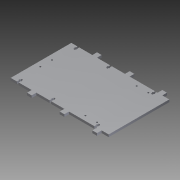
# Autodesk Inventor part: pieza central base superior
Saved by Autodesk Inventor 2012 SP1 (Build 160190100, 190)
## iProperties
Created: 2014-12-27
Part Number: pieza central base superior
Material: Default
Document SubType Name: Modeling
Designer: PRINCIPAL
Density: 1 g/cm^3
Author: PRINCIPAL
Autodesk Inventor part; units mm, degrees
ref_plane "YZ Plane" through (0, 0, 0) normal (1, 0, 0) x (0, 1, 0)
ref_plane "XZ Plane" through (0, 0, 0) normal (0, 1, 0) x (-1, 0, 0)
ref_plane "XY Plane" through (0, 0, 0) normal (0, 0, 1) x (1, 0, 0)
sketch "Boceto1" plane through (0, 0, 0) normal (0, 0, 1) x (1, 0, 0)
  line L0 (0, 0) -> (195, 0)
  line L1 (195, 0) -> (195, -130)
  line L2 (195, -130) -> (0, -130)
  line L3 (-15, 0) -> (-15, -130)
  line L4 (0, -130) -> (-15, -130)
  line L5 (0, 0) -> (-15, 0)
  dimension "d1" = 130
  constraints: 12 end point, 2 parallel, 2 perpendicular, 1 horizontal
  measures "d1" distance between parallel lines of L2 L0
extrude "Extrusión1" add sketch "Boceto1" along normal blind 5
sketch "Boceto2" plane through (0, 0, 5) normal (0, 0, 1) x (1, 0, 0)
  line L0 (-15, 0) -> (195, 0) projected
  line L1 (195, -130) -> (-15, -130) projected
  line L2 (30, 0) -> (40, 0)
  line L3 (100, 0) -> (110, 0)
  line L4 (170, 0) -> (180, 0)
  line L5 (170, -130) -> (180, -130)
  line L6 (100, -130) -> (110, -130)
  line L7 (30, -130) -> (40, -130)
  line L8 (40, 5) -> (40, 0)
  line L9 (40, -130) -> (40, -135)
  line L10 (30, -135) -> (30, -130)
  line L11 (30, 0) -> (30, 5)
  line L12 (110, 5) -> (110, 0)
  line L13 (110, -130) -> (110, -135)
  line L14 (100, -135) -> (100, -130)
  line L15 (100, 0) -> (100, 5)
  line L16 (180, 5) -> (180, 0)
  line L17 (180, -130) -> (180, -135)
  line L18 (170, -135) -> (170, -130)
  line L19 (170, 0) -> (170, 5)
  line L20 (30, 5) -> (30, 10)
  line L21 (40, 10) -> (40, 5)
  line L22 (100, 5) -> (100, 10)
  line L23 (110, 10) -> (110, 5)
  line L24 (170, 5) -> (170, 10)
  line L25 (180, 10) -> (180, 5)
  line L26 (40, -135) -> (40, -140)
  line L27 (30, -140) -> (30, -135)
  line L28 (110, -135) -> (110, -140)
  line L29 (100, -140) -> (100, -135)
  line L30 (180, -135) -> (180, -140)
  line L31 (170, -140) -> (170, -135)
  line L32 (170, 10) -> (180, 10)
  line L33 (30, 10) -> (40, 10)
  line L34 (100, 10) -> (110, 10)
  line L35 (180, -140) -> (170, -140)
  line L36 (110, -140) -> (100, -140)
  line L37 (40, -140) -> (30, -140)
  constraints: 72 end point, 27 perpendicular, 24 equal length, 12 point on line
extrude "Extrusión2" add sketch "Boceto2" against normal blind 5
sketch "Boceto3" plane through (0, 0, 5) normal (0, 0, 1) x (1, 0, 0)
  line L0 (195, 0) -> (195, -130) projected
  line L1 (180, 0) -> (195, 0) projected
  line L2 (-15, -130) -> (-15, 0) projected
  circle A0 centre (135, -120) radius 1.75
  circle A1 centre (160, -120) radius 1.75
  circle A2 centre (135, -10) radius 1.75
  circle A3 centre (160, -10) radius 1.75
  circle A4 centre (-4, -52.5) radius 1.75
  circle A5 centre (-4, -77.5) radius 1.75
  point P0 (30, 0)
  point P1 (30, -130)
  point P2 (0, 0)
  dimension "d20" = 3.5
  dimension "d21" = 3.5
  dimension "d22" = 3.5
  dimension "d23" = 3.5
  dimension "d24" = 3.5
  dimension "d25" = 3.5
  dimension "d26" = 25
  dimension "d27" = 25
  dimension "d28" = 25
  dimension "d29" = 10
  dimension "d30" = 10
  dimension "d31" = 150
  dimension "d32" = 150
  dimension "d33" = 52.5
  dimension "d34" = 199
  constraints: 6 centre point
  measures "d20" diameter of A0
  measures "d21" diameter of A1
  measures "d22" diameter of A2
  measures "d23" diameter of A3
  measures "d24" diameter of A4
  measures "d25" diameter of A5
  measures "d26" distance of A3.centre A2.centre
  measures "d27" distance of A1.centre A0.centre
  measures "d28" distance of A4.centre A5.centre
  measures "d29" vertical distance of A2.centre point (30, 0)
  measures "d30" vertical distance of point (30, -130) A0.centre
  measures "d31" distance from line of A0.centre L2
  measures "d32" distance from line of L2 A2.centre
  measures "d33" distance from line of A4.centre L1
  measures "d34" distance from line of L0 A4.centre
extrude "Extrusión3" cut sketch "Boceto3" against normal blind 10
sketch "Boceto4" plane through (0, 0, 5) normal (0, 0, 1) x (1, 0, 0)
  line L0 (-1.6674, -130.3426) -> (-1.6674, -125.4313)
  line L1 (1.8326, -130.3426) -> (-1.6674, -130.3426)
  line L2 (1.8326, -125.4313) -> (1.8326, -130.3426)
  line L3 (-1.6674, -125.4313) -> (-2.6674, -125.4313)
  line L4 (-2.6674, -123.0313) -> (-1.6674, -123.0313)
  line L5 (-1.6674, -123.0313) -> (-1.6674, -120.2573)
  line L6 (1.8326, -120.2573) -> (1.8326, -123.0313)
  line L7 (2.8326, -125.4313) -> (1.8326, -125.4313)
  line L8 (2.8326, -123.0313) -> (2.8326, -125.4313)
  line L9 (1.8326, -123.0313) -> (2.8326, -123.0313)
  line L10 (1.8326, -120.2573) -> (-1.6674, -120.2573)
  line L11 (-2.6674, -125.4313) -> (-2.6674, -123.0313)
  line L12 (167.9972, -120.715) -> (164.4972, -120.715)
  line L13 (167.9972, -120.715) -> (167.9972, -123.4891)
  line L14 (164.4972, -123.4891) -> (164.4972, -120.715)
  line L15 (167.9972, -123.4891) -> (168.9972, -123.4891)
  line L16 (168.9972, -123.4891) -> (168.9972, -125.8891)
  line L17 (163.4972, -125.8891) -> (163.4972, -123.4891)
  line L18 (164.4972, -125.8891) -> (163.4972, -125.8891)
  line L19 (168.9972, -125.8891) -> (167.9972, -125.8891)
  line L20 (163.4972, -123.4891) -> (164.4972, -123.4891)
  line L21 (164.4972, -130.8004) -> (164.4972, -125.8891)
  line L22 (167.9972, -130.8004) -> (164.4972, -130.8004)
  line L23 (167.9972, -125.8891) -> (167.9972, -130.8004)
  line L24 (71.7006, -120.3125) -> (68.2006, -120.3125)
  line L25 (71.7006, -120.3125) -> (71.7006, -123.0866)
  line L26 (68.2006, -123.0866) -> (68.2006, -120.3125)
  line L27 (71.7006, -123.0866) -> (72.7006, -123.0866)
  line L28 (72.7006, -123.0866) -> (72.7006, -125.4866)
  line L29 (67.2006, -125.4866) -> (67.2006, -123.0866)
  line L30 (68.2006, -125.4866) -> (67.2006, -125.4866)
  line L31 (72.7006, -125.4866) -> (71.7006, -125.4866)
  line L32 (67.2006, -123.0866) -> (68.2006, -123.0866)
  line L33 (68.2006, -130.3979) -> (68.2006, -125.4866)
  line L34 (71.7006, -130.3979) -> (68.2006, -130.3979)
  line L35 (71.7006, -125.4866) -> (71.7006, -130.3979)
  line L36 (1.8326, -9.3206) -> (-1.6674, -9.3206)
  line L37 (1.8326, -9.3206) -> (1.8326, -6.5466)
  line L38 (-1.6674, -6.5466) -> (-1.6674, -9.3206)
  line L39 (1.8326, -6.5466) -> (2.8326, -6.5466)
  line L40 (2.8326, -6.5466) -> (2.8326, -4.1466)
  line L41 (-2.6674, -4.1466) -> (-2.6674, -6.5466)
  line L42 (-1.6674, -4.1466) -> (-2.6674, -4.1466)
  line L43 (2.8326, -4.1466) -> (1.8326, -4.1466)
  line L44 (-2.6674, -6.5466) -> (-1.6674, -6.5466)
  line L45 (-1.6674, 0.7647) -> (-1.6674, -4.1466)
  line L46 (1.8326, 0.7647) -> (-1.6674, 0.7647)
  line L47 (1.8326, -4.1466) -> (1.8326, 0.7647)
  line L48 (168.9375, -3.8347) -> (167.9375, -3.8347)
  line L49 (167.9375, -3.8347) -> (167.9375, 1.0766)
  line L50 (167.9375, 1.0766) -> (164.4375, 1.0766)
  line L51 (167.9375, -6.2347) -> (168.9375, -6.2347)
  line L52 (167.9375, -9.0087) -> (167.9375, -6.2347)
  line L53 (164.4375, 1.0766) -> (164.4375, -3.8347)
  line L54 (164.4375, -3.8347) -> (163.4375, -3.8347)
  line L55 (163.4375, -3.8347) -> (163.4375, -6.2347)
  line L56 (163.4375, -6.2347) -> (164.4375, -6.2347)
  line L57 (164.4375, -6.2347) -> (164.4375, -9.0087)
  line L58 (167.9375, -9.0087) -> (164.4375, -9.0087)
  line L59 (168.9375, -6.2347) -> (168.9375, -3.8347)
  line L60 (72.7006, -6.4914) -> (72.7006, -4.0914)
  line L61 (72.7006, -4.0914) -> (71.7006, -4.0914)
  line L62 (71.7006, -6.4914) -> (72.7006, -6.4914)
  line L63 (71.7006, -4.0914) -> (71.7006, 0.8199)
  line L64 (71.7006, -9.2654) -> (71.7006, -6.4914)
  line L65 (71.7006, 0.8199) -> (68.2006, 0.8199)
  line L66 (68.2006, 0.8199) -> (68.2006, -4.0914)
  line L67 (71.7006, -9.2654) -> (68.2006, -9.2654)
  line L68 (68.2006, -6.4914) -> (68.2006, -9.2654)
  line L69 (68.2006, -4.0914) -> (67.2006, -4.0914)
  line L70 (67.2006, -4.0914) -> (67.2006, -6.4914)
  line L71 (67.2006, -6.4914) -> (68.2006, -6.4914)
  line L72 (170, 10) -> (170, 0) projected
  point P0 (0, 0)
  dimension "d37" = 3.5
  dimension "d38" = 3.5
  dimension "d39" = 3.5
  dimension "d45" = 2.0625
  constraints: 144 end point
  measures "d37" distance between parallel lines of L5 L6
  measures "d38" distance between parallel lines of L14 L13
  measures "d39" distance between parallel lines of L26 L25
  measures "d45" distance from line of L50.start L72
extrude "Extrusión4" cut sketch "Boceto4" against normal blind 10
